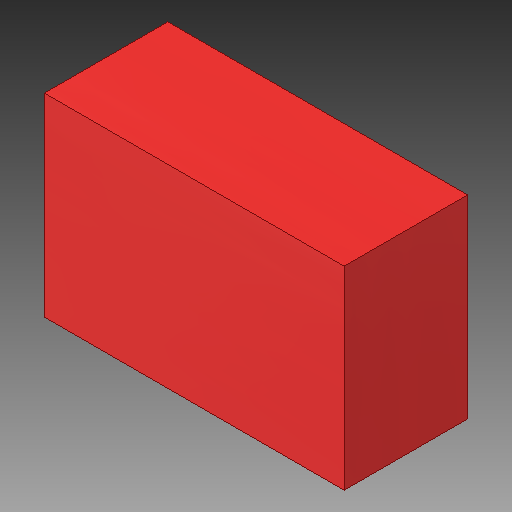
# Autodesk Inventor part: 回路2
Saved by Autodesk Inventor 2020 (Build 240168000, 168)
## iProperties
Part Number: 回路2
Material: 一般
Document SubType Name: Sheet Metal
Designer: 雪村
Density: 0.483516 g/cm^3
Appearance: 淡い赤
Mass: 55 g
Surface Area: 158.5 cm^2
Volume: 113.75 cm^3
Sheet Metal Rule: Default
Author: 雪村
Autodesk Inventor part; units mm, degrees
ref_plane "YZ Plane" through (0, 0, 0) normal (1, 0, 0) x (0, 1, 0)
ref_plane "XZ Plane" through (0, 0, 0) normal (0, 1, 0) x (-1, 0, 0)
ref_plane "XY Plane" through (0, 0, 0) normal (0, 0, 1) x (1, 0, 0)
sketch "スケッチ1" plane through (0, 0, 0) normal (0, 0, 1) x (1, 0, 0)
  line L0 (0, 0) -> (70, 0)
  line L1 (70, 0) -> (70, 55)
  line L2 (70, 55) -> (0, 55)
  line L3 (0, 55) -> (0, 0)
  dimension "d1" = 70
  dimension "d2" = 55
  constraints: 8 end point, 2 vertical, 1 horizontal
  measures "d1" distance of L2.end L1.end
  measures "d2" distance of L1.end L0.end
extrude "押し出し1" add sketch "スケッチ1" along normal blind 35
sketch "スケッチ2" plane through (0, 0, 0) normal (0, 0, -1) x (-1, 0, 0)
  line L0 (0, 0) -> (-70, 0) projected
  line L1 (0, 55) -> (0, 0) projected
  line L2 (-70, 55) -> (0, 55) projected
  line L3 (-70, 0) -> (-70, 55) projected
  line L4 (0, 0) -> (15, 0)
  line L5 (15, 0) -> (15, 55)
  line L6 (-70, 55) -> (0, 55) projected
  line L7 (15, 55) -> (0, 55)
  dimension "d5" = 15
  constraints: 6 end point, 2 horizontal, 1 vertical
  measures "d5" distance of L0.start L4.end
extrude "押し出し2" add sketch "スケッチ2" against normal blind 35 contours L1 L7 L5 L4
